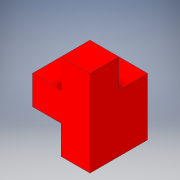
# Autodesk Inventor part: CubePart2
Saved by Autodesk Inventor 2019 (Build 230136000, 136)
## iProperties
Created: 2019-09-11
Part Number: CubePart2
Material: Generic
Document SubType Name: Modeling
Designer: IED8
Density: 1 g/cm^3
Appearance: Default
Author: IED8
Autodesk Inventor part; units mm, degrees
ref_plane "YZ Plane" through (0, 0, 0) normal (1, 0, 0) x (0, 1, 0)
ref_plane "XZ Plane" through (0, 0, 0) normal (0, 1, 0) x (-1, 0, 0)
ref_plane "XY Plane" through (0, 0, 0) normal (0, 0, 1) x (1, 0, 0)
sketch "Sketch1" plane through (0, 0, 0) normal (1, 0, 0) x (0, 1, 0)
  line L0 (0, 0) -> (0, -38.1)
  line L1 (0, -38.1) -> (57.15, -38.1)
  line L2 (57.15, -38.1) -> (57.15, -19.05)
  line L3 (57.15, -19.05) -> (38.1, -19.05)
  line L4 (38.1, -19.05) -> (38.1, 0)
  line L5 (38.1, 0) -> (0, 0)
  dimension "d0" = 38.1
  dimension "d1" = 57.15
  dimension "d2" = 19.05
  constraints: 12 end point, 5 perpendicular, 1 vertical
  measures "d0" distance of L0.start L0.end
  measures "d1" distance of L0.end L1.end
  measures "d2" distance of L2.end L3.end
extrude "Extrusion1" add sketch "Sketch1" along normal blind 19.05
sketch "Sketch2" plane through (0, 0, 0) normal (-1, 0, 0) x (0, 0, 1)
  line L0 (-19.05, 38.1) -> (0, 38.1) projected
  line L1 (-19.05, 38.1) -> (-19.05, 19.05)
  line L2 (-19.05, 19.05) -> (0, 19.05)
  line L3 (0, 38.1) -> (0, 0) projected
  line L4 (0, 19.05) -> (0, 38.1)
  line L5 (0, 38.1) -> (-19.05, 38.1)
  dimension "d5" = 19.05
  constraints: 8 end point, 2 perpendicular, 1 collinear, 1 vertical
  measures "d5" distance of L0.start L1.end
extrude "Extrusion2" add sketch "Sketch2" along normal blind 19.05
sketch "Sketch3" plane through (0, 57.15, -19.05) normal (0, 0, 1) x (1, 0, 0)
  line L0 (0, 0) -> (19.05, 0) projected
  line L1 (0, 0) -> (19.05, 0)
  line L2 (19.05, 0) -> (19.05, -18.7133)
  line L3 (19.05, -57.15) -> (19.05, 0) projected
  line L4 (0, -57.15) -> (0, 0) projected
  line L5 (0, 0) -> (0, -18.7133)
  line L6 (0, -19.05) -> (19.05, -19.05) projected
  line L7 (19.05, -19.05) -> (0, -19.05)
  constraints: 8 end point, 2 collinear, 2 point on line
extrude "Extrusion3" cut sketch "Sketch3" against normal blind 19.05
sketch "Sketch4" plane through (0, 38.1, -38.1) normal (0, 1, 0) x (1, 0, 0)
  line L0 (0, -38.1) -> (0, -19.05) projected
  line L1 (0, -19.05) -> (19.05, -19.05)
  line L2 (19.05, -38.1) -> (19.05, 0) projected
  line L3 (19.05, -19.05) -> (19.05, -38.1)
  line L4 (19.05, -38.1) -> (0, -38.1)
  line L5 (-19.05, -38.1) -> (19.05, -38.1) projected
  line L6 (0, -19.05) -> (-19.05, -19.05) projected
  line L7 (0, -19.05) -> (0, -38.1)
  constraints: 8 end point, 2 collinear, 1 midpoint, 1 perpendicular
extrude "Extrusion4" add sketch "Sketch4" along normal blind 19.05
body "Solid1"
